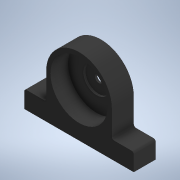
# Autodesk Inventor part: sg_motor_mount
Saved by Autodesk Inventor 2022 (Build 260153000, 153)
## iProperties
Created: 2022-10-06
Part Number: sg_motor_mount
Material: Generic
Document SubType Name: Modeling
Designer: janni
Density: 1 g/cm^3
Appearance: Rubber - Black
Author: janni
Autodesk Inventor part; units mm, degrees
ref_plane "YZ Plane" through (0, 0, 0) normal (1, 0, 0) x (0, 1, 0)
ref_plane "XZ Plane" through (0, 0, 0) normal (0, 1, 0) x (-1, 0, 0)
ref_plane "XY Plane" through (0, 0, 0) normal (0, 0, 1) x (1, 0, 0)
sketch "Sketch2" plane through (0, 0, 0) normal (0, 0, 1) x (1, 0, 0)
  line L0 (25, 8) -> (25, 0)
  line L1 (25, 0) -> (-25, 0)
  line L2 (-25, 0) -> (-25, 8)
  line L3 (0, -7) -> (0, 42) projected
  arc A0 (15, 20) -> (-15, 20) centre (0, 20) ccw
  line L4 (0, 42) -> (0, -7) projected
  line L5 (-15, 20) -> (-15, 8)
  line L6 (15, 20) -> (15, 8)
  line L7 (-35, 0) -> (35, 0) projected
  line L8 (-25, 8) -> (-15, 8)
  line L9 (15, 8) -> (25, 8)
  point P0 (0, 0)
  dimension "d4" = 50
  dimension "d6" = 20
  dimension "d7" = 30
  dimension "d8" = 8
  dimension "d9" = 8
  constraints: 14 end point, 6 perpendicular, 3 parallel, 2 horizontal, 2 point on circle, 2 tangent, 1 centre point, 1 collinear, 1 point on line, 1 other
  measures "d4" distance between parallel lines of L0 L2
  measures "d6" distance from line of L1 A0.centre
  measures "d7" diameter of A0
  measures "d8" distance between parallel lines of L1 L8
  measures "d9" distance between parallel lines of L1 L9
extrude "Extrusion2" add sketch "Sketch2" against normal blind 10
sketch "Sketch3" plane through (0, 0, 0) normal (0, 0, 1) x (1, 0, 0)
  arc A0 (15, 20) -> (-15, 20) centre (0, 20) ccw projected
  circle A1 centre (0, 20) radius 13.05
  point P0 (0, 0)
  dimension "d12" = 26.1
  constraints: 1 centre point, 1 coincident
  measures "d12" diameter of A1
extrude "Extrusion3" cut sketch "Sketch3" against normal blind 8
sketch "Sketch4" plane through (0, 20, -8) normal (0, 0, 1) x (1, 0, 0)
  circle A0 centre (0, 0) radius 6.05
  point P0 (0, -20)
  dimension "d15" = 12.1
  constraints: 1 centre point
  measures "d15" diameter of A0
extrude "Extrusion4" cut sketch "Sketch4" against normal blind 1
sketch "Sketch5" plane through (0, 20, -9) normal (0, 0, 1) x (1, 0, 0)
  circle A0 centre (0, 0) radius 1.75
  point P0 (0, -20)
  dimension "d18" = 3.5
  constraints: 1 centre point
  measures "d18" diameter of A0
extrude "Extrusion5" cut sketch "Sketch5" against normal blind 1
sketch "Sketch6" plane through (-25, 0, 0) normal (0, -1, 0) x (1, 0, 0)
  circle A0 centre (5, -5) radius 2
  circle A1 centre (45, -5) radius 2
  line L0 (25, -12) -> (25, 2) projected
  line L1 (50, -10) -> (0, -10) projected
  point P0 (25, 0)
  dimension "d21" = 4
  dimension "d22" = 40
  dimension "d23" = 5
  constraints: 2 centre point, 1 equal radius, 1 symmetric about line
  measures "d21" diameter of A0
  measures "d22" distance of A1.centre A0.centre
  measures "d23" distance from line of L1 A0.centre
extrude "Extrusion6" cut sketch "Sketch6" against normal blind 6
fillet "Fillet1" radius 1 4 edges at (-15, 8, -5) (-25, 8, -5) (15, 8, -5) (25, 8, -5)
body "Solid2"
